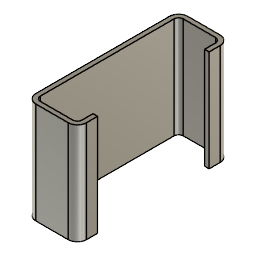
RC-150×50×20×4.5 (Autodesk Fusion 360 design; units mm, degrees)
Autodesk Fusion 360 part; units mm, degrees
sketch "スケッチ1" plane through (0, 0, 0) normal (0, 0, 1) x (1, 0, 0)
sketch "スケッチ2" plane through (0, 0, 0) normal (0, 0, 1) x (1, 0, 0)
  line L0 (427.9082, -74.1289) -> (427.9082, -206.1289)
  line L1 (423.4082, -74.1289) -> (423.4082, -206.1289)
  line L2 (464.4082, -215.1289) -> (432.4082, -215.1289)
  line L3 (432.4082, -210.6289) -> (464.4082, -210.6289)
  arc A0 (423.4082, -206.1289) -> (432.4082, -215.1289) centre (432.4082, -206.1289) ccw
  arc A1 (427.9082, -206.1289) -> (432.4082, -210.6289) centre (432.4082, -206.1289) ccw
  arc A2 (464.4082, -215.1289) -> (473.4082, -206.1289) centre (464.4082, -206.1289) ccw
  line L4 (468.9082, -206.1289) -> (468.9082, -195.1289)
  line L5 (473.4082, -206.1289) -> (473.4082, -195.1289)
  arc A3 (464.4082, -210.6289) -> (468.9082, -206.1289) centre (464.4082, -206.1289) ccw
  line L6 (473.4082, -195.1289) -> (468.9082, -195.1289)
  line L7 (432.4082, -69.6289) -> (464.4082, -69.6289)
  line L8 (432.4082, -65.1289) -> (464.4082, -65.1289)
  arc A4 (432.4082, -65.1289) -> (423.4082, -74.1289) centre (432.4082, -74.1289) ccw
  arc A5 (432.4082, -69.6289) -> (427.9082, -74.1289) centre (432.4082, -74.1289) ccw
  arc A6 (473.4082, -74.1289) -> (464.4082, -65.1289) centre (464.4082, -74.1289) ccw
  arc A7 (468.9082, -74.1289) -> (464.4082, -69.6289) centre (464.4082, -74.1289) ccw
  line L9 (468.9082, -85.1289) -> (473.4082, -85.1289)
  line L10 (468.9082, -74.1289) -> (468.9082, -85.1289)
  line L11 (473.4082, -74.1289) -> (473.4082, -85.1289)
  point P0 (423.4082, -65.1289)
extrude "押し出し1" add sketch "スケッチ2" along normal blind 100
